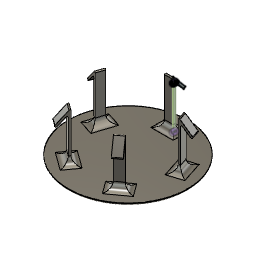
4-inch-can-light-blank-cover-v2 (Autodesk Fusion 360 design; units mm, degrees)
Autodesk Fusion 360 part; units mm, degrees
sketch "Sketch1" plane through (0, 0, 0) normal (0, 1, 0) x (1, 0, 0)
  circle A0 centre (0, 0) radius 70
  dimension "d1" = 140
  constraint coincident A0.centre origin
  measures "d1" diameter of A0
extrude "Extrude1" add sketch "Sketch1" along normal blind 3
sketch "Sketch2" plane through (0, 3, 0) normal (0, 1, 0) x (-1, 0, 0)
  circle A0 centre (0, 0) radius 70
  line L0 (-4.19584, -51.193533) -> (5.80416, -51.193533)
  line L1 (5.80416, -51.193533) -> (5.80416, -48.793533)
  line L2 (5.80416, -48.793533) -> (-4.19584, -48.793533)
  line L3 (-4.19584, -48.793533) -> (-4.19584, -51.193533)
  arc A1 (5.80416, -49.661975) -> (-4.19584, -49.823638) centre (0, 0) ccw construction
  line L4 (47.391357, -19.810153) -> (50.481527, -10.299588)
  line L5 (48.198991, -9.557947) -> (45.108821, -19.068512)
  line L6 (50.481527, -10.299588) -> (48.198991, -9.557947)
  line L7 (45.108821, -19.068512) -> (47.391357, -19.810153)
  line L8 (33.48531, 38.950185) -> (25.39514, 44.828038)
  line L9 (23.984455, 42.886397) -> (32.074625, 37.008544)
  line L10 (25.39514, 44.828038) -> (23.984455, 42.886397)
  line L11 (32.074625, 37.008544) -> (33.48531, 38.950185)
  line L12 (-26.696297, 43.882691) -> (-34.786467, 38.004839)
  line L13 (-33.375783, 36.063198) -> (-25.285613, 41.94105)
  line L14 (-34.786467, 38.004839) -> (-33.375783, 36.063198)
  line L15 (-25.285613, 41.94105) -> (-26.696297, 43.882691)
  line L16 (-49.984529, -11.82919) -> (-46.894359, -21.339756)
  line L17 (-44.611823, -20.598115) -> (-47.701993, -11.08755)
  line L18 (-46.894359, -21.339756) -> (-44.611823, -20.598115)
  line L19 (-47.701993, -11.08755) -> (-49.984529, -11.82919)
  point P0 (46.08851, -19.386832)
  point P1 (49.024929, -9.82631)
  point P2 (32.680106, 37.841917)
  point P3 (24.494913, 43.588981)
  point P4 (-25.891094, 42.774423)
  point P5 (-33.88624, 36.765782)
  point P6 (-48.681682, -11.40587)
  point P7 (-45.437761, -20.866478)
  dimension "d4" = 100
  dimension "d5" = 2.4
  dimension "d6" = 10
  dimension "d8" = 360
  constraint coincident A0.centre A1.centre
  constraint horizontal L0
  constraint perpendicular L0 L1
  constraint parallel L0 L2
  constraint parallel L1 L3
  measures "d4" diameter of A1
extrude "Extrude2" add sketch "Sketch2" along normal blind 50 contours L0 L1 L2 L3 | L4 L5 L6 L7 | L8 L9 L10 L11 | L12 L13 L14 L15 | L16 L17 L18 L19 picked at (-0.862507, -49.593533) picked at (48.690625, -13.222563) picked at (27.621635, 42.22154) picked at (-31.149288, 38.669696) picked at (-47.16357, -17.922354)
sketch "Sketch3" plane through (4.19584, 0, 0) normal (1, 0, 0) x (0, 0, -1)
  line L0 (48.793533, 3) -> (51.193533, 3)
  line L1 (51.193533, 3) -> (51.193533, 53)
  line L2 (51.193533, 53) -> (48.793533, 53)
  line L3 (48.793533, 53) -> (48.793533, 3)
  line L4 (51.193533, 53) -> (61.21972, 41.051256)
  line L5 (61.21972, 41.051256) -> (63.058227, 42.593946)
  line L6 (48.793533, 59.593946) -> (63.058227, 42.593946)
  line L7 (48.793533, 53) -> (48.793533, 59.593946)
  line L8 (48.793533, 3) -> (51.193533, 3)
  line L9 (51.193533, 3) -> (51.193533, 53)
  line L10 (51.193533, 53) -> (48.793533, 53)
  line L11 (48.793533, 53) -> (48.793533, 3)
  dimension "d11" = 2.4
  dimension "d12" = 40
  dimension "d13" = 90
  dimension "d16" = 17
  constraint perpendicular L4 L5
  constraint parallel L4 L6
  measures "d12" angle of L1 L4
  measures "d13" angle of L2 L7
sketch "Sketch6" plane through (1.296586, 0, -3.990481) normal (0.309017, 0, -0.951057) x (-0.951057, 0, -0.309017)
  line L0 (48.793533, 3) -> (51.193533, 3)
  line L1 (51.193533, 3) -> (51.193533, 53)
  line L2 (51.193533, 53) -> (48.793533, 53)
  line L3 (48.793533, 53) -> (48.793533, 3)
  line L4 (48.793533, 59.593946) -> (63.058227, 42.593946)
  line L5 (51.193533, 53) -> (48.793533, 53)
  line L6 (51.193533, 53) -> (61.21972, 41.051256)
  line L7 (51.193533, 53) -> (48.793533, 53)
  line L8 (48.793533, 53) -> (48.793533, 59.593946)
  line L9 (61.21972, 41.051256) -> (63.058227, 42.593946)
  dimension "d25" = 2.4
  dimension "d26" = 90
  dimension "d27" = 17
  constraint perpendicular L6 L9
  constraint parallel L4 L6
  measures "d26" angle of L5 L8
sketch "Sketch7" plane through (-3.394506, 0, -2.466253) normal (-0.809017, 0, -0.587785) x (-0.587785, 0, 0.809017)
  line L0 (48.793533, 3) -> (51.193533, 3)
  line L1 (51.193533, 3) -> (51.193533, 53)
  line L2 (51.193533, 53) -> (48.793533, 53)
  line L3 (48.793533, 53) -> (48.793533, 3)
  line L4 (48.793533, 59.593946) -> (63.058227, 42.593946)
  line L5 (51.193533, 53) -> (48.793533, 53)
  line L6 (51.193533, 53) -> (61.21972, 41.051256)
  line L7 (51.193533, 53) -> (48.793533, 53)
  line L8 (48.793533, 53) -> (48.793533, 59.593946)
  line L9 (61.21972, 41.051256) -> (63.058227, 42.593946)
  dimension "d28" = 2.4
  dimension "d29" = 90
  dimension "d30" = 17
  constraint perpendicular L6 L9
  constraint parallel L4 L6
  measures "d29" angle of L5 L8
sketch "Sketch8" plane through (-3.394506, 0, 2.466253) normal (-0.809017, 0, 0.587785) x (0.587785, 0, 0.809017)
  line L0 (48.793533, 3) -> (51.193533, 3)
  line L1 (51.193533, 3) -> (51.193533, 53)
  line L2 (51.193533, 53) -> (48.793533, 53)
  line L3 (48.793533, 53) -> (48.793533, 3)
  line L4 (48.793533, 59.593946) -> (63.058227, 42.593946)
  line L5 (51.193533, 53) -> (48.793533, 53)
  line L6 (51.193533, 53) -> (61.21972, 41.051256)
  line L7 (51.193533, 53) -> (48.793533, 53)
  line L8 (48.793533, 53) -> (48.793533, 59.593946)
  line L9 (61.21972, 41.051256) -> (63.058227, 42.593946)
  dimension "d31" = 2.4
  dimension "d32" = 90
  dimension "d33" = 17
  constraint perpendicular L6 L9
  constraint parallel L4 L6
  measures "d32" angle of L5 L8
sketch "Sketch9" plane through (1.296586, 0, 3.990481) normal (0.309017, 0, 0.951057) x (0.951057, 0, -0.309017)
  line L0 (48.793533, 3) -> (51.193533, 3)
  line L1 (51.193533, 3) -> (51.193533, 53)
  line L2 (51.193533, 53) -> (48.793533, 53)
  line L3 (48.793533, 53) -> (48.793533, 3)
  line L4 (48.793533, 59.593946) -> (63.058227, 42.593946)
  line L5 (51.193533, 53) -> (48.793533, 53)
  line L6 (51.193533, 53) -> (61.21972, 41.051256)
  line L7 (51.193533, 53) -> (48.793533, 53)
  line L8 (48.793533, 53) -> (48.793533, 59.593946)
  line L9 (61.21972, 41.051256) -> (63.058227, 42.593946)
  dimension "d34" = 2.4
  dimension "d35" = 90
  dimension "d36" = 17
  constraint perpendicular L6 L9
  constraint parallel L4 L6
  measures "d35" angle of L5 L8
extrude "Extrude4" add sketch "Sketch3" against normal blind 10 contours L2 L4 L5 L6 L7 L10 picked at (54.348431, 51.729297)
extrude "Extrude5" add sketch "Sketch6" against normal blind 10 contours L2 L4 L5 L6 L7 L8 L9 picked at (54.348431, 51.729297)
extrude "Extrude6" add sketch "Sketch7" against normal blind 10 contours L2 L4 L5 L6 L7 L8 L9 picked at (54.348431, 51.729297)
extrude "Extrude7" add sketch "Sketch8" against normal blind 10 contours L2 L4 L5 L6 L7 L8 L9 picked at (54.348431, 51.729297)
extrude "Extrude8" add sketch "Sketch9" against normal blind 10 contours L2 L4 L5 L6 L7 L8 L9 picked at (54.348431, 51.729297)
fillet "Fillet1" radius 8 10 edges at (-29.440225, 3, 41.889111) (30.741382, 3, 40.943765) (48.439444, 3, -16.584473) (-0.80416, 3, -51.193533) (-48.936442, 3, -15.05487) (29.330698, 3, 39.002124) (-28.02954, 3, 39.94747) (46.156908, 3, -15.842832) (-0.80416, 3, -48.793533) (-46.653906, 3, -14.31323)
fillet "Fillet2" radius 8 10 edges at (-24.689798, 3, 43.857217) (34.081125, 3, 37.034018) (-49.340259, 3, -9.928767) (45.753091, 3, -20.968935) (-5.80416, 3, -49.993533) (-46.250089, 3, -19.439333) (4.19584, 3, -49.993533) (48.843261, 3, -11.45837) (25.990955, 3, 42.911871) (-32.779967, 3, 37.979365)
fillet "Fillet3" radius 1 10 edges at (-46.653906, 59.593946, -14.31323) (-48.936442, 53, -15.05487) (-28.02954, 59.593946, 39.94747) (-29.440225, 53, 41.889111) (29.330698, 59.593946, 39.002124) (30.741382, 53, 40.943765) (46.156908, 59.593946, -15.842832) (48.439444, 53, -16.584473) (-0.80416, 59.593946, -48.793533) (-0.80416, 53, -51.193533)
fillet "Fillet4" radius 1 10 edges at (-0.80416, 42.593946, -63.058227) (-0.80416, 41.051256, -61.21972) (-60.220436, 42.593946, -18.721262) (-58.471913, 41.051256, -18.153133) (-36.414117, 42.593946, 51.48785) (-35.33347, 41.051256, 50.000467) (37.715274, 42.593946, 50.542504) (36.634627, 41.051256, 49.055121) (59.723438, 42.593946, -20.250865) (57.974915, 41.051256, -19.682735)
fillet "Fillet5" radius 2.4 1 edges at (-65.262914, 0, 25.31308)
equation "d1 = cover_outer_diameter"
equation "d2 = cover_height"
equation "d4 = claw_diameter"
equation "d5 = claw_thickness"
equation "d6 = claw_width"
equation "d9 = claw_height"
equation "d11 = claw_thickness"
equation "d12 = claw_angle"
equation "d16 = claw_diag_length"
equation "claw_angle = 40 deg"
equation "claw_thickness = 2.4 mm"
equation "claw_diag_length = 17 mm"
equation "claw_width = 10 mm"
equation "cover_outer_diameter = 140 mm"
equation "cover_height = 3 mm"
equation "claw_diameter = 100 mm"
equation "claw_height = 50 mm"
equation "d25 = claw_thickness"
equation "d27 = claw_diag_length"
equation "d28 = claw_thickness"
equation "d30 = claw_diag_length"
equation "d31 = claw_thickness"
equation "d33 = claw_diag_length"
equation "d34 = claw_thickness"
equation "d36 = claw_diag_length"
equation "d37 = -claw_width"
equation "d39 = -claw_width"
equation "d41 = -claw_width"
equation "d43 = -claw_width"
equation "d45 = -claw_width"
